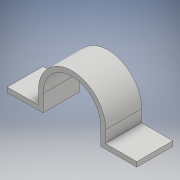
# Autodesk Inventor part: Hange
Saved by Autodesk Inventor 2017 (Build 210142000, 142)
## iProperties
Created: 2017-11-16
Part Number: Hange
Material: Generic
Document SubType Name: Modeling
Designer: DesignPC02
Density: 1 g/cm^3
Appearance: Default
Author: DesignPC02
Autodesk Inventor part; units mm, degrees
ref_plane "YZ Plane" through (0, 0, 0) normal (1, 0, 0) x (0, 1, 0)
ref_plane "XZ Plane" through (0, 0, 0) normal (0, 1, 0) x (-1, 0, 0)
ref_plane "XY Plane" through (0, 0, 0) normal (0, 0, 1) x (1, 0, 0)
sketch "Sketch3" plane through (0, 0, 0) normal (0, 1, 0) x (-1, 0, 0)
  arc A0 (11.9985, -0.1919) -> (-11.9985, -0.1919) centre (0, 0) ccw
  line L0 (11.9985, -0.1919) -> (12, -7.1919)
  line L1 (12, -7.1919) -> (26.9985, -7.4066)
  line L2 (-11.9985, -0.1919) -> (-11.9985, -7.2992)
  line L3 (-11.9985, -7.2992) -> (-26.9985, -7.2992)
  line L4 (-26.9985, -5.2992) -> (-13.9985, -5.2992)
  line L5 (-13.9985, -5.2992) -> (-13.9985, -0.2073)
  arc A1 (13.9985, -0.207) -> (-13.9985, -0.2073) centre (0, 0) ccw
  line L6 (13.9985, -0.207) -> (13.9996, -5.2203)
  line L7 (13.9996, -5.2203) -> (26.9985, -5.4064)
  line L8 (-26.9985, -5.2992) -> (-26.9985, -7.2992)
  line L9 (26.9985, -5.4064) -> (26.9985, -7.4066)
  dimension "d25" = 24
  dimension "d26" = 7
  dimension "d27" = 15
  dimension "d28" = 15
  dimension "d29" = 2
  constraints: 20 end point, 4 point on circle, 2 centre point, 2 perpendicular, 2 vertical, 1 coincident, 1 parallel, 4 other
  measures "d25" diameter of A0
  measures "d26" distance of L0.start L0.end
  measures "d27" distance of L0.end L1.end
  measures "d28" distance of L2.end L3.end
  measures "d29" radial gap between concentric circles of A0 A1
extrude "Extrusion3" add sketch "Sketch3" along normal blind 15
body "Solid2"
